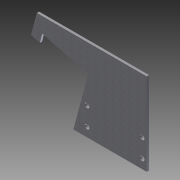
# Autodesk Inventor part: plate_metal_hook
Saved by Autodesk Inventor 2011 (Build 150239000, 239)
## iProperties
Created: 2013-01-17
Part Number: plate_metal_hook
Document SubType Name: Modeling
Designer: Christopher
Density: 1 g/cm^3
Author: Christopher
Autodesk Inventor part; units mm, degrees
ref_plane "YZ Plane" through (0, 0, 0) normal (1, 0, 0) x (0, 1, 0)
ref_plane "XZ Plane" through (0, 0, 0) normal (0, 1, 0) x (-1, 0, 0)
ref_plane "XY Plane" through (0, 0, 0) normal (0, 0, 1) x (1, 0, 0)
sketch "Sketch1" plane through (0, 0, 0) normal (0, 0, 1) x (1, 0, 0)
  line L0 (62.419, -58.294) -> (151.319, -58.294)
  line L1 (62.419, -58.294) -> (49.719, -58.294)
  line L2 (49.719, -58.294) -> (70.1368, 17.906)
  line L3 (70.1368, 17.906) -> (6.6368, 34.9207)
  line L4 (6.6368, 34.9207) -> (3.2338, 22.2207)
  line L5 (3.2338, 22.2207) -> (-9.0335, 25.5077)
  line L6 (-9.0335, 25.5077) -> (-0.8615, 56.006)
  line L7 (151.319, 56.006) -> (151.319, -58.294)
  line L8 (151.319, 56.006) -> (-0.8615, 56.006)
  point P0 (0, 0)
  point P1 (145.018, -45.594)
  point P2 (145.018, -20.194)
  point P3 (68.818, -20.194)
  point P4 (68.818, -45.594)
  dimension "d3" = 88.9
  dimension "d9" = 76.2
  dimension "d10" = 25.4
  dimension "d11" = 12.7
  dimension "d22" = 12.7
  dimension "d23" = 75
  dimension "d24" = 76.2
  dimension "d25" = 63.5
  dimension "d26" = 12.7
  dimension "d27" = 12.7
  dimension "d29" = 114.3
  constraints: 18 end point, 7 perpendicular, 2 horizontal alignment, 2 vertical alignment, 1 horizontal
  measures "d3" distance of L0.start L0.end
  measures "d9" distance of point (145.018, -45.594) point (68.818, -45.594)
  measures "d10" distance of point (68.818, -45.594) point (68.818, -20.194)
  measures "d11" distance from line of L0 point (68.818, -45.594)
  measures "d22" distance of L0.start L1.end
  measures "d23" angle of L0 L2
  measures "d24" vertical distance of L1.end L2.end
  measures "d25" horizontal distance of L2.end L3.end
  measures "d26" vertical distance of L3.end L4.end
  measures "d27" distance of L4.end L5.end
  measures "d29" distance of L7.start L0.end
extrude "Extrusion1" add sketch "Sketch1" against normal blind 3.175
hole "Hole1" at (145.018, -45.594, 0) at (145.018, -20.194, 0) at (68.818, -20.194, 0) at (68.818, -45.594, 0) direction (0, 0, -1) diameter 6.35 depth 25.4 tip angle 118
fillet "Fillet1" radius 12.7 2 edges at (70.1368, 17.906, -1.5875) (6.6368, 34.9207, -1.5875)
body "Solid1"
